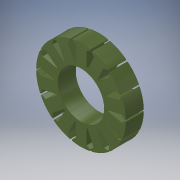
# Autodesk Inventor part: stator
Saved by Autodesk Inventor 2019.4 (Build 234330000, 330)
## iProperties
Created: 2019-10-01
Part Number: stator
Material: Generic
Document SubType Name: Modeling
Designer: cdi
Density: 1 g/cm^3
Appearance: Dark Olive
Author: cdi
Autodesk Inventor part; units mm, degrees
ref_plane "YZ Plane" through (0, 0, 0) normal (1, 0, 0) x (0, 1, 0)
ref_plane "XZ Plane" through (0, 0, 0) normal (0, 1, 0) x (-1, 0, 0)
ref_plane "XY Plane" through (0, 0, 0) normal (0, 0, 1) x (1, 0, 0)
sketch "Sketch1" plane through (0, 0, 0) normal (0, 0, 1) x (1, 0, 0)
  arc A0 (5.0505, 24.4845) -> (-5.0505, 24.4845) centre (0, 0) ccw
  line L0 (0, 0) -> (0, 32.4048)
  line L1 (-3, 0) -> (-3, 22.8035)
  line L2 (-4.0404, 24.6713) -> (-4.0404, 32.6515)
  line L3 (3, 0) -> (3, 22.8035)
  line L4 (4.0404, 24.6713) -> (4.0404, 32.6515)
  arc A1 (-5, 14.1421) -> (5, 14.1421) centre (0, 0) ccw
  arc A2 (3, 14.4568) -> (-3, 14.4568) centre (0, 0) ccw
  arc A3 (-3, 22.8035) -> (-5.0505, 22.4386) centre (0, 0) ccw
  arc A4 (5.0505, 22.4386) -> (3, 22.8035) centre (0, 0) ccw
  line L5 (-5, 0) -> (-5, 14.1421)
  line L6 (-5.0505, 22.4386) -> (-5.0505, 24.4845)
  line L7 (5, 0) -> (5, 14.1421)
  line L8 (5.0505, 22.4386) -> (5.0505, 24.4845)
  dimension "d0" = 50
  dimension "d9" = 6
  dimension "d10" = 3
  constraints: 18 end point, 12 parallel, 12 point on circle, 5 centre point, 2 coincident, 2 point on line, 1 vertical
  measures "d0" diameter of A0
  measures "d9" distance between parallel lines of L1 L3
  measures "d10" distance between parallel lines of L3 L0
extrude "Extrusion1" add sketch "Sketch1" along normal blind 10
sketch "Sketch2" plane through (0, 0, 10) normal (0, 0, 1) x (1, 0, 0)
  arc A0 (5.0505, 22.4386) -> (3, 22.8035) centre (0, 0) ccw projected
  line L0 (3, 22.8035) -> (5.0505, 23.9845)
  line L1 (5.0505, 22.4386) -> (5.0505, 24.4845) projected
  dimension "d11" = 0.5
  constraints: 2 end point
  measures "d11" distance of L1.end L0.end
extrude "Extrusion2" cut sketch "Sketch2" against normal blind 10
mirror "Mirror1" about plane through (0, 0, 0) normal (1, 0, 0) of "Extrusion2"
pattern_circular "Circular Pattern1" count 14 over 360 about axis through (0, 0, -10) along (0, 0, 1) of "Extrusion1", "Extrusion2", "Mirror1"
sketch "Sketch3" plane through (0, 0, 10) normal (0, 0, 1) x (1, 0, 0)
  arc A0 (3, 14.4568) -> (-3, 14.4568) centre (0, 0) ccw projected
  circle A1 centre (0, 0) radius 14.7648
  circle A2 centre (0, 0) radius 13
  dimension "d17" = 26
  constraints: 2 coincident, 1 centre point, 3 other
  measures "d17" diameter of A2
extrude "Extrusion3" add sketch "Sketch3" against normal blind 10
equation "\"d10\" = 0.5 * d9"
equation "\"d3\" = 0.5 * d2"
equation "\"d5\" = 0.5 * d4"
equation "\"d2\" = 8"
equation "\"d4\" = 10"
body "Solid1"
